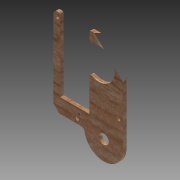
# Autodesk Inventor part: p1
Saved by Autodesk Inventor 2015 (Build 190159000, 159)
## iProperties
Created: 2016-02-03
Part Number: p1
Material: Generic
Document SubType Name: Modeling
Designer: david
Density: 1 g/cm^3
Appearance: Birch - Natural Polished
Mass: 14.4344 g
Surface Area: 101.883 cm^2
Volume: 14.4344 cm^3
Author: david
Autodesk Inventor part; units mm, degrees
ref_plane "YZ Plane" through (0, 0, 0) normal (1, 0, 0) x (0, 1, 0)
ref_plane "XZ Plane" through (0, 0, 0) normal (0, 1, 0) x (-1, 0, 0)
ref_plane "XY Plane" through (0, 0, 0) normal (0, 0, 1) x (1, 0, 0)
sketch "Sketch1" plane through (0, 0, 0) normal (0, 1, 0) x (-1, 0, 0)
  line L0 (20, 45) -> (-20, 45)
  line L1 (-20, 45) -> (-20, -45)
  line L2 (-20, -45) -> (20, -45)
  line L3 (20, -45) -> (20, 45)
  line L4 (20, 45) -> (-20, -45) construction
  line L5 (-20, 45) -> (20, -45) construction
  arc A0 (-20, -45) -> (20, -45) centre (0, -45) ccw
  line L6 (20, -45) -> (52, -45)
  line L7 (52, -45) -> (52, 45)
  line L8 (52, 45) -> (20, 45)
  line L9 (20, 45) -> (20, -45)
  point P0 (0, 0)
  dimension "d0" = 40
  dimension "d1" = 90
  dimension "d7" = 32
  dimension "d8" = 90
  constraints: 20 end point, 4 parallel, 3 midpoint, 2 horizontal, 2 perpendicular, 2 point on circle, 1 centre point
  measures "d0" distance of L2.end L1.end
  measures "d1" distance of L1.end L0.end
  measures "d7" distance of L8.end L7.end
  measures "d8" distance of L7.end L6.end
extrude "Extrusion1" add sketch "Sketch1" along normal blind 3.6
sketch "Sketch2" plane through (0, 3.6, 0) normal (0, 1, 0) x (1, 0, 0)
  arc A0 (20, 45) -> (-20, 45) centre (0, 45) ccw projected
  circle A1 centre (0, 45) radius 5.15
  point P0 (0, 0)
  dimension "d4" = 10.3
  constraints: 1 centre point, 1 coincident
  measures "d4" diameter of A1
extrude "Extrusion2" cut sketch "Sketch2" against normal blind 3.6
fillet "Fillet1" radius 4 4 edges at (-20, 1.8, -45) (-52, 1.8, -45) (-52, 1.8, 45) (20, 1.8, 45)
sketch "Sketch3" plane through (0, 0, 0) normal (0, -1, 0) x (1, 0, 0)
  line L0 (-48, 45) -> (16, 45) projected
  line L1 (-45, 45) -> (-15, 45)
  line L2 (-15, 45) -> (-15, -30)
  line L3 (-15, -30) -> (-45, -30)
  line L4 (-45, -30) -> (-45, 45)
  line L5 (-52, -41) -> (-52, 41) projected
  circle A0 centre (-5, 20) radius 16.25
  line L6 (20, 41) -> (20, -45) projected
  point P0 (0, 0)
  dimension "d10" = 30
  dimension "d11" = 75
  dimension "d12" = 7
  dimension "d13" = 32.5
  dimension "d14" = 25
  dimension "d15" = 25
  constraints: 8 end point, 2 parallel, 1 centre point, 1 horizontal, 1 perpendicular, 1 point on line
  measures "d10" distance of L2.end L3.end
  measures "d11" distance of L1.end L2.end
  measures "d12" distance between parallel lines of L5 L4
  measures "d13" diameter of A0
  measures "d14" distance from line of L6 A0.centre
  measures "d15" distance from line of L0 A0.centre
extrude "Extrusion3" cut sketch "Sketch3" against normal blind 10
fillet "Fillet2" radius 2 3 edges at (-15, 1.8, 45) (-15, 1.8, 32.8087) (-15, 1.8, 7.1913)
sketch "Sketch4" plane through (0, 0, 0) normal (0, -1, 0) x (1, 0, 0)
  circle A0 centre (-27.5, -40.5) radius 1.625
  circle A1 centre (15.5, 40.5) radius 1.625
  circle A2 centre (15.5, -19.5) radius 1.625
  line L0 (20, 41) -> (20, -45) projected
  line L1 (-13, 45) -> (16, 45) projected
  line L2 (-23.6643, -45) -> (-48, -45) projected
  line L3 (-52, -41) -> (-52, 41) projected
  point P0 (0, 0)
  dimension "d19" = 3.25
  dimension "d20" = 3.25
  dimension "d21" = 3.25
  dimension "d22" = 4.5
  dimension "d23" = 4.5
  dimension "d24" = 4.5
  dimension "d25" = 60
  dimension "d26" = 4.5
  dimension "d27" = 24.5
  constraints: 3 centre point
  measures "d19" diameter of A0
  measures "d20" diameter of A1
  measures "d21" diameter of A2
  measures "d22" distance from line of L0 A1.centre
  measures "d23" distance from line of L1 A1.centre
  measures "d24" distance from line of L0 A2.centre
  measures "d25" distance between centres of A1 A2
  measures "d26" distance from line of L2 A0.centre
  measures "d27" distance from line of L3 A0.centre
extrude "Extrusion4" cut sketch "Sketch4" against normal blind 10
sketch "Sketch5" plane through (0, 3.6, 0) normal (0, 1, 0) x (1, 0, 0)
  circle A0 centre (-48, -40) radius 1.575
  line L0 (-52, 41) -> (-52, -41) projected
  line L1 (-13, -45) -> (16, -45) projected
  point P0 (0, 0)
  dimension "d30" = 3.15
  dimension "d31" = 4
  dimension "d32" = 5
  constraints: 1 centre point
  measures "d30" diameter of A0
  measures "d31" distance from line of L0 A0.centre
  measures "d32" distance from line of L1 A0.centre
extrude "Extrusion5" cut sketch "Sketch5" against normal blind 10
body "Solid1"
